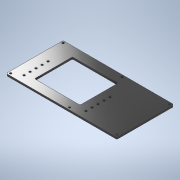
# Autodesk Inventor part: Sole_frame
Saved by Autodesk Inventor 2020.4 (Build 244396000, 396)
## iProperties
Part Number: Sole_frame
Material: GFRP
Document SubType Name: Modeling
Designer: Masato Kubotera
Density: 1.75 g/cm^3
Appearance: 低 光沢 - 黒
Description: GFRP T3
Mass: 61.6656 g
Surface Area: 261.936 cm^2
Volume: 35.2375 cm^3
Author: Masato Kubotera
Autodesk Inventor part; units mm, degrees
ref_plane "YZ Plane" through (0, 0, 0) normal (1, 0, 0) x (0, 1, 0)
ref_plane "XZ Plane" through (0, 0, 0) normal (0, 1, 0) x (-1, 0, 0)
ref_plane "XY Plane" through (0, 0, 0) normal (0, 0, 1) x (1, 0, 0)
sketch "スケッチ1" plane through (0, 0, 0) normal (0, 0, 1) x (1, 0, 0)
  line L0 (-96.735, 64.25) -> (78.265, 64.25)
  line L1 (78.265, 64.25) -> (78.265, -25.75)
  line L2 (78.265, -25.75) -> (-96.735, -25.75)
  line L3 (-96.735, -25.75) -> (-96.735, 64.25)
  line L4 (-96.735, 64.25) -> (78.265, -25.75) construction
  line L5 (78.265, 64.25) -> (-96.735, -25.75) construction
  line L6 (-96.735, 19.25) -> (78.265, 19.25) construction
  line L7 (-96.735, 0) -> (78.265, 0) construction
  line L8 (-80, 4.75) -> (-80, -4.75) construction
  circle A0 centre (-80, -4.75) radius 1.6
  line L9 (0, 64.25) -> (0, -25.75) construction
  line L10 (18, -4.75) -> (18, 4.75) construction
  circle A1 centre (18, -4.75) radius 1.6
  circle A2 centre (-80, 4.75) radius 1.6
  circle A3 centre (18, 4.75) radius 1.6
  line L11 (74.765, -22.25) -> (-93.235, -22.25) construction
  line L12 (-93.235, -22.25) -> (-93.235, 60.75) construction
  line L13 (-93.235, 60.75) -> (74.765, 60.75) construction
  line L14 (74.765, 60.75) -> (74.765, -22.25) construction
  line L15 (74.765, -22.25) -> (-93.235, 60.75) construction
  line L16 (-93.235, -22.25) -> (74.765, 60.75) construction
  circle A4 centre (-93.235, 60.75) radius 1.6
  circle A5 centre (0, 60.75) radius 1.6
  circle A6 centre (74.765, 60.75) radius 1.6
  circle A7 centre (-93.235, -22.25) radius 1.6
  circle A8 centre (0, -22.25) radius 1.6
  circle A9 centre (74.765, -22.25) radius 1.6
  line L17 (15, 12.5) -> (21, 12.5) construction
  line L18 (21, 12.5) -> (21, -12.5) construction
  line L19 (21, -12.5) -> (15, -12.5) construction
  line L20 (15, -12.5) -> (15, 12.5) construction
  line L21 (15, 12.5) -> (21, -12.5) construction
  line L22 (21, 12.5) -> (15, -12.5) construction
  line L23 (-83, 12.5) -> (-77, 12.5) construction
  line L24 (-77, 12.5) -> (-77, -12.5) construction
  line L25 (-77, -12.5) -> (-83, -12.5) construction
  line L26 (-83, -12.5) -> (-83, 12.5) construction
  line L27 (-83, 12.5) -> (-77, -12.5) construction
  line L28 (-77, 12.5) -> (-83, -12.5) construction
  line L29 (-67, 49.25) -> (5, 49.25)
  line L30 (5, 49.25) -> (5, -10.75)
  line L31 (5, -10.75) -> (-67, -10.75)
  line L32 (-67, -10.75) -> (-67, 49.25)
  line L33 (-67, 49.25) -> (5, -10.75) construction
  line L34 (5, 49.25) -> (-67, -10.75) construction
  line L35 (-83, -3) -> (-83, 22) construction
  line L36 (-83, 22) -> (-77, 22) construction
  line L37 (-77, 22) -> (-77, -3) construction
  line L38 (-77, -3) -> (-83, -3) construction
  circle A10 centre (-80, 14.25) radius 1.6
  circle A11 centre (-80, 4.75) radius 1.6
  line L39 (15, 22) -> (21, 22) construction
  line L40 (15, -3) -> (15, 22) construction
  line L41 (21, -3) -> (15, -3) construction
  line L42 (21, 22) -> (21, -3) construction
  circle A12 centre (18, 4.75) radius 1.6
  circle A13 centre (18, 14.25) radius 1.6
  line L43 (-83, 6.5) -> (-83, 31.5) construction
  line L44 (-83, 31.5) -> (-77, 31.5) construction
  line L45 (-77, 31.5) -> (-77, 6.5) construction
  line L46 (-77, 6.5) -> (-83, 6.5) construction
  circle A14 centre (-80, 23.75) radius 1.6
  circle A15 centre (-80, 14.25) radius 1.6
  line L47 (15, 31.5) -> (21, 31.5) construction
  line L48 (15, 6.5) -> (15, 31.5) construction
  line L49 (21, 6.5) -> (15, 6.5) construction
  line L50 (21, 31.5) -> (21, 6.5) construction
  circle A16 centre (18, 14.25) radius 1.6
  circle A17 centre (18, 23.75) radius 1.6
  circle A18 centre (-80, -14.25) radius 1.6
  line L51 (-77, -22) -> (-83, -22) construction
  line L52 (-83, -22) -> (-83, 3) construction
  line L53 (-77, 3) -> (-77, -22) construction
  line L54 (15, -22) -> (15, 3) construction
  circle A19 centre (18, -14.25) radius 1.6
  line L55 (21, -22) -> (15, -22) construction
  line L56 (21, 3) -> (21, -22) construction
  point P0 (0, 0)
  point P1 (-9.235, 19.25)
  point P2 (-80, 0)
  point P3 (18, 0)
  point P4 (-31, 19.25)
  dimension "d0" = 175
  dimension "d1" = 90
  dimension "d2" = 25.75
  dimension "d3" = 3.2
  dimension "d4" = 9.5
  dimension "d5" = 9.5
  dimension "d6" = 3.2
  dimension "d9" = 3.5
  dimension "d10" = 3.5
  dimension "d11" = 3.2
  dimension "d13" = 3.2
  dimension "d15" = 3.2
  dimension "d16" = 78.265
  dimension "d17" = 6
  dimension "d18" = 25
  dimension "d19" = 21
  dimension "d20" = 6
  dimension "d21" = 25
  dimension "d22" = 104
  dimension "d23" = 15
  dimension "d24" = 15
  dimension "d25" = 10
  dimension "d26" = 10
  dimension "d57" = 9.5
  dimension "d64" = 9.5
  constraints: 114 end point, 20 centre point, 14 midpoint, 10 parallel, 10 point on line, 7 perpendicular, 5 horizontal, 5 symmetric about line, 4 coincident, 4 vertical, 2 collinear, 69 other
  measures "d0" distance of L1.end L2.end
  measures "d1" distance of L0.end L1.end
  measures "d2" distance of L2.end L7.start
  measures "d3" diameter of A0
  measures "d4" distance of L8.start L8.end
  measures "d5" distance of L10.start L10.end
  measures "d6" diameter of A1
  measures "d9" horizontal distance of L0.start L12.end
  measures "d10" horizontal distance of L0.start L12.end
  measures "d11" diameter of A4
  measures "d13" diameter of A5
  measures "d15" diameter of A6
  measures "d16" distance of L0.end L9.start
  measures "d17" distance of L18.end L19.end
  measures "d18" distance of L17.end L18.end
  measures "d19" horizontal distance of L17.end point (0, 0)
  measures "d20" distance of L24.end L25.end
  measures "d21" distance of L23.end L24.end
  measures "d22" distance of L18.end L25.end
  measures "d23" distance between parallel lines of L29 L0
  measures "d24" distance between parallel lines of L2 L31
  measures "d25" distance between parallel lines of L32 L24
  measures "d26" distance between parallel lines of L20 L30
  measures "d57" distance of L25.end L35.start
  measures "d64" distance of A0.centre A18.centre
extrude "押し出し1" add sketch "スケッチ1" along normal blind 3
fillet "フィレット1" radius 2 4 edges at (-96.735, 64.25, 1.5) (78.265, 64.25, 1.5) (78.265, -25.75, 1.5) (-96.735, -25.75, 1.5)
fillet "フィレット2" radius 2 4 edges at (-67, 49.25, 1.5) (-67, -10.75, 1.5) (5, -10.75, 1.5) (5, 49.25, 1.5)
equation "\"d3\" = d6"
equation "\"d4\" = d5"
equation "\"d10\" = d9"
equation "\"d11\" = d3"
equation "\"d13\" = d11"
equation "\"d15\" = d13"
equation "\"d20\" = d17"
equation "\"d21\" = d18"
